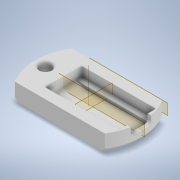
# Autodesk Inventor part: hmmb
Saved by Autodesk Inventor 2021 (Build 250183000, 183)
## iProperties
Created: 2020-07-09
Part Number: hmmb
Material: Generic
Document SubType Name: Modeling
Designer: andre
Density: 1 g/cm^3
Appearance: Default
Author: andre
## iProperties of the stored document _3DPrint.ipt
Created: 2020-07-09
Part Number: _3DPrint
Material: Generic
Document SubType Name: Modeling
Designer: andre
Density: 1 g/cm^3
Appearance: Default
Author: andre
Autodesk Inventor part; units mm, degrees
ref_plane "YZ Plane" through (0, 0, 0) normal (1, 0, 0) x (0, 1, 0)
ref_plane "XZ Plane" through (0, 0, 0) normal (0, 1, 0) x (-1, 0, 0)
ref_plane "XY Plane" through (0, 0, 0) normal (0, 0, 1) x (1, 0, 0)
sketch "Sketch1" plane through (0, 0, 0) normal (0, 1, 0) x (-1, 0, 0)
  circle A0 centre (0, 0) radius 26
  dimension "d0" = 52
  constraints: 1 centre point
  measures "d0" diameter of A0
extrude "Extrusion1" add sketch "Sketch1" along normal blind 8
chamfer "Chamfer2" distance 1.6 angle 45 1 edges at (26, 0, 0)
sketch "Sketch2" plane through (0, 8, 0) normal (0, 1, 0) x (1, 0, 0)
  line L0 (-12.4, -8.99) -> (23.96, -8.99)
  line L1 (23.96, -8.99) -> (23.96, 8.99)
  line L2 (23.96, 8.99) -> (-12.4, 8.99)
  line L3 (-12.4, 8.99) -> (-12.4, -8.99)
  point P0 (0, 0)
  dimension "d5" = 36.36
  dimension "d6" = 17.98
  dimension "d7" = 8.99
  dimension "d8" = 12.4
  constraints: 8 end point, 2 parallel, 1 horizontal, 1 perpendicular
  measures "d5" distance of L2.end L1.end
  measures "d6" distance of L1.end L0.end
  measures "d7" distance from line of point (0, 0) L2
  measures "d8" distance from line of point (0, 0) L3
extrude "Extrusion2" cut sketch "Sketch2" against normal blind 4.8
sketch "Sketch3" plane through (23.96, 8, -8.99) normal (-1, 0, 0) x (0, 0, 1)
  line L0 (4, 0) -> (13.98, 0)
  line L1 (13.98, 0) -> (13.98, -3.8)
  line L2 (13.98, -3.8) -> (4, -3.8)
  line L3 (4, -3.8) -> (4, 0)
  line L4 (0, 0) -> (17.98, 0) projected
  line L5 (0, -4.8) -> (17.98, -4.8) projected
  line L6 (0, 0) -> (0, -4.8) projected
  line L7 (17.98, 0) -> (17.98, -4.8) projected
  point P0 (8.99, -8)
  dimension "d11" = 0
  dimension "d14" = 4
  dimension "d44" = 4
  dimension "d47" = 1
  constraints: 8 end point, 2 parallel, 1 horizontal, 1 perpendicular
  measures "d11" distance between parallel lines of L4 L0
  measures "d14" distance between parallel lines of L7 L1
  measures "d44" distance between parallel lines of L6 L3
  measures "d47" distance between parallel lines of L5 L2
extrude "Extrusion3" cut sketch "Sketch3" against normal through all contours L0 L1 L2 L3
ref_plane "Work Plane1" through (-12.4, 8, 0) normal (0, 0, 1) x (1, 0, 0)
sketch "Sketch7" plane through (0, 3.2, 0) normal (0, 1, 0) x (1, 0, 0)
  line L0 (-12.4, 6.35) -> (23.16, 6.35)
  line L1 (23.16, 6.35) -> (23.16, -6.35)
  line L2 (23.16, -6.35) -> (-12.4, -6.35)
  line L3 (-12.4, -6.35) -> (-12.4, 6.35)
  line L4 (36.4, 0) -> (-36.4, 0) projected
  line L5 (-12.4, -8.99) -> (-12.4, 8.99) projected
  line L6 (23.96, -8.99) -> (-12.4, -8.99) projected
  point P0 (0, 0)
  dimension "d28" = 12.7
  dimension "d29" = 35.56
  dimension "d30" = 6.35
  dimension "d31" = 0
  dimension "d79" = 2.64
  constraints: 8 end point, 2 parallel, 1 horizontal, 1 perpendicular
  measures "d28" distance of L0.end L1.end
  measures "d29" distance between parallel lines of L1 L3
  measures "d30" distance between parallel lines of L4 L0
  measures "d31" distance between parallel lines of L5 L3
  measures "d79" distance between parallel lines of L6 L2
extrude "Extrusion5" cut sketch "Sketch7" against normal blind 1.6
sketch "Sketch4" plane through (0, 8, 0) normal (0, 1, 0) x (1, 0, 0)
  circle A0 centre (-21, 0) radius 2.8
  arc A1 (25.5167, 4.99) -> (25.5167, -4.99) centre (0, 0) ccw projected
  point P0 (24.6995, 8.12)
  point P1 (24.6995, -8.12)
  dimension "d17" = 5.6
  dimension "d23" = 21
  constraints: 1 centre point
  measures "d17" diameter of A0
  measures "d23" distance of A0.centre A1.centre
extrude "Extrusion4" cut sketch "Sketch4" against normal blind 5.2
fillet "Fillet4" radius 1 1 edges at (-23.8, 8, 0)
pattern_circular "Circular Pattern2" count 5 over 240 about axis through (0, 8, 0) along (0, 1, 0) of "Extrusion4", "Fillet4" both ways yes
chamfer "Chamfer3" distance 1.5 distance2 5 1 edges at (-12.4, 1.6, 0) measured on face at (-12.4, 2.1, 0)
fillet "Fillet7" radius 0.8 4 edges at (23.96, 5.6, -8.99) (23.96, 5.6, 8.99) (-12.4, 5.6, 8.99) (-12.4, 5.6, -8.99) curvature continuous yes
sketch "Sketch12" plane through (0, 0, 0) normal (0, -1, 0) x (1, 0, 0)
  line L0 (12.3547, 12.0872) -> (12.3547, -12.0872) construction
  line L1 (12.3547, -12.0872) -> (-12.3547, -12.0872) construction
  line L2 (-12.3547, -12.0872) -> (-12.3547, 12.0872) construction
  line L3 (-12.3547, 12.0872) -> (12.3547, 12.0872) construction
  spline S0 degree 2 poles (-6.9887, 9.9266) (-7, 9.452) (-6.4915, 8.8644) (-5.9379, 8.7062) knots 0 0 0 1 2 2 2
  line L4 (-5.9379, 8.7062) -> (-3.3503, 7.8023)
  line L5 (-3.3503, 7.8023) -> (-3.3503, 2.6949)
  line L6 (-3.3503, 2.6949) -> (-5.9605, 1.8023)
  spline S1 degree 2 poles (-5.9605, 1.8023) (-6.5028, 1.6441) (-7, 1.0452) (-6.9887, 0.548) knots 0 0 0 1 2 2 2
  spline S2 degree 2 poles (-6.9887, 0.548) (-6.9887, 0.0057) (-6.3672, -0.661) (-5.8701, -0.6723) knots 0 0 0 1 2 2 2
  spline S3 degree 2 poles (-5.8701, -0.6723) (-5.7006, -0.6723) (-5.3503, -0.5932) (-5.113, -0.5141) knots 0 0 0 1 2 2 2
  line L7 (-5.113, -0.5141) -> (5.678, 3.4633)
  spline S4 degree 2 poles (5.678, 3.4633) (6.3672, 3.7232) (7, 4.5819) (6.9887, 5.2599) knots 0 0 0 1 2 2 2
  spline S5 degree 2 poles (6.9887, 5.2599) (7, 5.9153) (6.3446, 6.7853) (5.6667, 7.0226) knots 0 0 0 1 2 2 2
  line L8 (5.6667, 7.0226) -> (-5.113, 10.9887)
  spline S6 degree 2 poles (-5.113, 10.9887) (-5.339, 11.0791) (-5.7232, 11.1582) (-5.8701, 11.1582) knots 0 0 0 1 2 2 2
  spline S7 degree 2 poles (-5.8701, 11.1582) (-6.3898, 11.1469) (-6.9887, 10.4915) (-6.9887, 9.9266) knots 0 0 0 1 2 2 2
  line L9 (-1.4181, 7.226) -> (4.4237, 5.3051)
  line L10 (4.4237, 5.3051) -> (4.4237, 5.2373)
  line L11 (4.4237, 5.2373) -> (-1.4181, 3.2938)
  line L12 (-1.4181, 3.2938) -> (-1.4181, 7.226)
  spline S8 degree 2 poles (-6.9887, -3.6667) (-6.9887, -4.2429) (-6.3333, -4.8757) (-5.7232, -4.887) knots 0 0 0 1 2 2 2
  line L13 (-5.7232, -4.887) -> (-1.2486, -4.887)
  line L14 (-1.2486, -4.887) -> (-1.2486, -9.7006)
  spline S9 degree 2 poles (-1.2486, -9.7006) (-1.2486, -10.1864) (-0.7288, -10.7627) (-0.2542, -10.774) knots 0 0 0 1 2 2 2
  spline S10 degree 2 poles (-0.2542, -10.774) (0.209, -10.7627) (0.7288, -10.1864) (0.7401, -9.7006) knots 0 0 0 1 2 2 2
  line L15 (0.7401, -9.7006) -> (0.7401, -4.887)
  line L16 (0.7401, -4.887) -> (4.774, -4.887)
  line L17 (4.774, -4.887) -> (4.774, -10.1977)
  spline S11 degree 2 poles (4.774, -10.1977) (4.774, -10.6949) (5.3164, -11.3051) (5.8023, -11.3164) knots 0 0 0 1 2 2 2
  spline S12 degree 2 poles (5.8023, -11.3164) (6.2768, -11.3051) (6.8305, -10.7062) (6.8305, -10.1977) knots 0 0 0 1 2 2 2
  line L18 (6.8305, -10.1977) -> (6.8305, -3.6667)
  spline S13 degree 2 poles (6.8305, -3.6667) (6.8305, -3.0904) (6.1638, -2.4463) (5.565, -2.435) knots 0 0 0 1 2 2 2
  line L19 (5.565, -2.435) -> (-5.7232, -2.435)
  spline S14 degree 2 poles (-5.7232, -2.435) (-6.3333, -2.4463) (-6.9887, -3.0904) (-6.9887, -3.6667) knots 0 0 0 1 2 2 2
  point P0 (0, 0)
  dimension "d80" = 24.1744
  dimension "d81" = 12.0872
  dimension "d82" = 24.7094
  dimension "d83" = 12.3547
  constraints: 2 other
  measures "d80" distance between parallel lines of L1 L3
  measures "d81" distance from line of point (0, 0) L1
  measures "d82" distance between parallel lines of L2 L0
  measures "d83" distance from line of point (0, 0) L2
extrude "Extrusion9" cut sketch "Sketch12" against normal blind 1
sketch "Sketch13" plane through (0, 0, 0) normal (0, -1, 0) x (1, 0, 0)
  line L0 (-14.251, 6.9467) -> (-14.251, -6.9467) construction
  line L1 (-14.251, -6.9467) -> (-20.3478, -6.9467) construction
  line L2 (-20.3478, -6.9467) -> (-20.3478, 6.9467) construction
  line L3 (-20.3478, 6.9467) -> (-14.251, 6.9467) construction
  line L4 (-36.4, 0) -> (36.4, 0) projected
  spline S0 degree 2 poles (-19.8075, 1.843) (-19.8034, 1.6135) (-19.5297, 1.3438) (-19.2962, 1.3398) knots 0 0 0 1 2 2 2
  line L5 (-19.2962, 1.3398) -> (-15.363, 1.3398)
  spline S1 degree 2 poles (-15.363, 1.3398) (-15.0973, 1.3438) (-14.7954, 1.6457) (-14.7913, 1.9195) knots 0 0 0 1 2 2 2
  spline S2 degree 2 poles (-14.7913, 1.9195) (-14.7913, 2.0725) (-14.8678, 2.3502) (-14.9846, 2.5233) knots 0 0 0 1 2 2 2
  line L6 (-14.9846, 2.5233) -> (-15.6529, 3.4895)
  spline S3 degree 2 poles (-15.6529, 3.4895) (-15.7374, 3.6063) (-15.9186, 3.711) (-16.0353, 3.711) knots 0 0 0 1 2 2 2
  spline S4 degree 2 poles (-16.0353, 3.711) (-16.2004, 3.7069) (-16.3976, 3.5097) (-16.3976, 3.3527) knots 0 0 0 1 2 2 2
  spline S5 degree 2 poles (-16.3976, 3.3527) (-16.3976, 3.2762) (-16.3574, 3.1514) (-16.3091, 3.0829) knots 0 0 0 1 2 2 2
  line L7 (-16.3091, 3.0829) -> (-15.8099, 2.3704)
  line L8 (-15.8099, 2.3704) -> (-15.8099, 2.3502)
  line L9 (-15.8099, 2.3502) -> (-19.2962, 2.3502)
  spline S6 degree 2 poles (-19.2962, 2.3502) (-19.5297, 2.3462) (-19.8034, 2.0725) (-19.8075, 1.843) knots 0 0 0 1 2 2 2
  spline S7 degree 2 poles (-19.8075, -1.2271) (-19.8075, -1.3881) (-19.6706, -1.6014) (-19.5095, -1.682) knots 0 0 0 1 2 2 2
  line L10 (-19.5095, -1.682) -> (-16.0232, -3.4855)
  spline S8 degree 2 poles (-16.0232, -3.4855) (-15.834, -3.5862) (-15.5562, -3.6787) (-15.4234, -3.6787) knots 0 0 0 1 2 2 2
  spline S9 degree 2 poles (-15.4234, -3.6787) (-15.1617, -3.6747) (-14.8678, -3.3406) (-14.8678, -3.0709) knots 0 0 0 1 2 2 2
  line L11 (-14.8678, -3.0709) -> (-14.8678, -0.5507)
  spline S10 degree 2 poles (-14.8678, -0.5507) (-14.8678, -0.3655) (-15.0852, -0.132) (-15.2704, -0.132) knots 0 0 0 1 2 2 2
  spline S11 degree 2 poles (-15.2704, -0.132) (-15.4556, -0.132) (-15.673, -0.3655) (-15.677, -0.5507) knots 0 0 0 1 2 2 2
  line L12 (-15.677, -0.5507) -> (-15.677, -2.6522)
  line L13 (-15.677, -2.6522) -> (-15.6971, -2.6522)
  line L14 (-15.6971, -2.6522) -> (-19.0707, -0.8486)
  spline S12 degree 2 poles (-19.0707, -0.8486) (-19.1513, -0.8043) (-19.3042, -0.7601) (-19.3928, -0.7601) knots 0 0 0 1 2 2 2
  spline S13 degree 2 poles (-19.3928, -0.7601) (-19.5699, -0.7641) (-19.8034, -1.0097) (-19.8075, -1.2271) knots 0 0 0 1 2 2 2
  point P0 (0, 0)
  dimension "d79" = 2.64
  dimension "d86" = 13.8935
  dimension "d87" = 6.9467
  constraints: 2 other
  measures "d86" distance between parallel lines of L1 L3
  measures "d87" distance between parallel lines of L4 L1
extrude "Extrusion10" cut sketch "Sketch13" against normal blind 2
fillet "Fillet9" radius 2 2 edges at (24.7383, 4.2, -4.99) (24.7383, 4.2, 4.99) curvature continuous yes
ref_plane "Work Plane3" through (-11.6, 8, -13.99) normal (0, 0, 1) x (1, 0, 0)
sketch "Sketch15" plane through (-11.6, 8, -13.99) normal (0, 0, 1) x (1, 0, 0)
  line L0 (-19.6997, 7.6359) -> (45.418, 7.6359)
  line L1 (45.418, 7.6359) -> (45.418, -14.4832)
  line L2 (45.418, -14.4832) -> (-19.6997, -14.4832)
  line L3 (-19.6997, -14.4832) -> (-19.6997, 7.6359)
  point P0 (11.6, -8)
  constraints: 8 end point, 2 parallel, 1 horizontal, 1 perpendicular
extrude "Extrusion11" cut sketch "Sketch15" against normal blind 15
mirror "Mirror5" about plane through (-12.4, 8, 0) normal (0, 0, 1) of "Extrusion11"
ref_plane "Work Plane4" through (2.6, 3.1, 6.35) normal (1, 0, 0) x (0, 0, -1)
equation "\"d7\" = 0.5 * d6"
equation "\"d44\" = d14"
equation "\"d30\" = 0.5 * d28"
equation "\"d81\" = 0.5 * d80"
equation "\"d83\" = 0.5 * d82"
equation "\"d24\" = 0.5 * d6"
body "Solid1"
